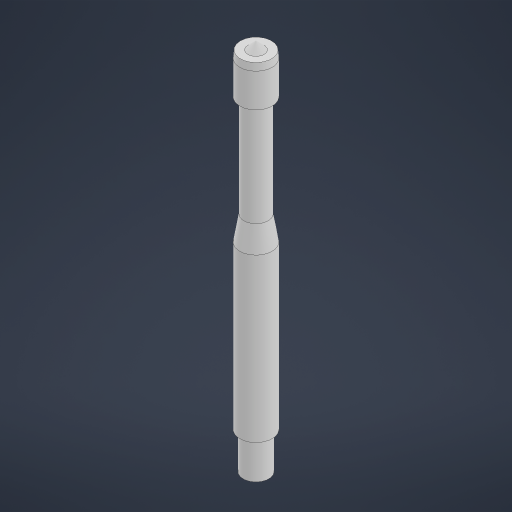
# Autodesk Inventor part: DORMER_SPU4908_M8SpiralFl_TAP
Saved by Autodesk Inventor 2024.3 (Build 283343000, 343)
## iProperties
Created: 2024-06-20
Part Number: DORMER_SPU4908_M8SpiralFl_TAP
Material: Generic
Document SubType Name: Modeling
Designer: fablabadmin
Density: 1 g/cm^3
Appearance: Default
Author: fablabadmin
Autodesk Inventor part; units mm, degrees
ref_plane "YZ Plane" through (0, 0, 0) normal (1, 0, 0) x (0, 1, 0)
ref_plane "XZ Plane" through (0, 0, 0) normal (0, 1, 0) x (-1, 0, 0)
ref_plane "XY Plane" through (0, 0, 0) normal (0, 0, 1) x (1, 0, 0)
sketch "Sketch1" plane through (0, 0, 0) normal (0, 0, 1) x (1, 0, 0)
  line L0 (-4.8, 0) -> (0.8, 0) construction
  line L1 (-3.15, 0) -> (-3.15, 9)
  line L2 (-3.15, 9) -> (-4, 9)
  line L3 (-4, 9) -> (-4, 49)
  line L4 (-4, 49) -> (-3, 55)
  line L5 (-3, 55) -> (-3, 80)
  line L6 (-3, 80) -> (-4, 80)
  line L7 (-4, 80) -> (-4, 88.25)
  line L8 (-4, 88.25) -> (-3.8469, 90)
  line L9 (-3.8469, 90) -> (-2, 90)
  line L10 (-2, 90) -> (0, 92)
  line L11 (0, 92) -> (0, 0)
  line L12 (-3.15, 0) -> (0, 0)
  dimension "d1" = 92
  dimension "d16" = 45
  dimension "d18" = 3.75
  dimension "d19" = 12
  dimension "d20" = 37
  dimension "d21" = 43
  dimension "d22" = 5
  dimension "d23" = 2
  dimension "d29" = 9
  dimension "d31" = 6.3
  dimension "d32" = 8
  dimension "d33" = 6
  dimension "d34" = 8
  constraints: 24 end point, 4 perpendicular, 2 vertical, 1 collinear, 1 horizontal, 1 parallel, 1 point on line
  measures "d1" distance of L11.end L10.end
  measures "d16" angle of L9 L10
  measures "d18" vertical distance of L7.end L10.end
  measures "d19" vertical distance of L6.end L10.end
  measures "d20" vertical distance of L4.end L10.end
  measures "d21" vertical distance of L3.end L10.end
  measures "d22" angle of L7 L8
  measures "d23" distance from line of L10.end L9
  measures "d29" distance of L1.start L1.end
  measures "d31" diameter of L1 L11
  measures "d32" diameter of L3 L11
  measures "d33" diameter of L5 L11
  measures "d34" diameter of L7 L11
revolve "Revolution3" add sketch "Sketch1" angle 360 about axis through (0, 92, 0) along (0, -1, 0)
body "Solid3"
